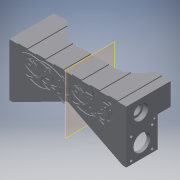
# Autodesk Inventor part: Crossmount
Saved by Autodesk Inventor 2016 (Build 200138000, 138)
## iProperties
Created: 2016-07-16
Part Number: Crossmount
Material: Generic
Document SubType Name: Modeling
Designer: Scott
Density: 1 g/cm^3
Appearance: Default
Author: Scott
Autodesk Inventor part; units mm, degrees
(part 1 of 2)
ref_plane "YZ Plane" through (0, 0, 0) normal (1, 0, 0) x (0, 1, 0)
ref_plane "XZ Plane" through (0, 0, 0) normal (0, 1, 0) x (-1, 0, 0)
ref_plane "XY Plane" through (0, 0, 0) normal (0, 0, 1) x (1, 0, 0)
sketch "Sketch1" plane through (0, 0, 0) normal (0, 0, 1) x (1, 0, 0)
  circle A0 centre (0, 0) radius 4 projected
  circle A1 centre (-152.4, 0) radius 4 projected
  circle A2 centre (0, 0) radius 10.16
  circle A3 centre (-152.4, 0) radius 10.16
  point P0 (0, 0)
  dimension "d0" = 20.32
  dimension "d1" = 20.32
  constraints: 2 centre point, 2 coincident
  measures "d0" diameter of A2
  measures "d1" diameter of A3
extrude "Extrusion1" add sketch "Sketch1" against normal blind 25.4
sketch "Sketch2" plane through (0, 0, 0) normal (0, 0, 1) x (1, 0, 0)
  circle A0 centre (-152.4, 0) radius 10.16 projected
  circle A1 centre (0, 0) radius 10.16 projected
  line L0 (10.16, -10.16) -> (-162.56, -10.16)
  line L1 (-162.56, -10.16) -> (-162.56, 10.16)
  line L2 (-162.56, 10.16) -> (10.16, 10.16)
  line L3 (10.16, 10.16) -> (10.16, -10.16)
  point P0 (0, 0)
  constraints: 8 end point, 2 parallel, 1 horizontal, 1 perpendicular
extrude "Extrusion2" add sketch "Sketch2" along normal blind 38.1
sketch "Sketch3" plane through (-162.56, -10.16, 0) normal (-1, 0, 0) x (0, 0, 1)
  circle A0 centre (18.605, 8.132) radius 4 projected
  line L0 (-0.445, -10.918) -> (37.655, -10.918)
  line L1 (37.655, -10.918) -> (37.655, 27.182)
  line L2 (37.655, 27.182) -> (-0.445, 27.182)
  line L3 (-0.445, 27.182) -> (-0.445, -10.918)
  line L4 (-0.445, -10.918) -> (37.655, 27.182) construction
  line L5 (37.655, -10.918) -> (-0.445, 27.182) construction
  point P0 (0, 10.16)
  dimension "d6" = 38.1
  dimension "d7" = 38.1
  constraints: 12 end point, 2 midpoint, 2 parallel, 1 horizontal, 1 perpendicular
  measures "d6" distance of L2.end L1.end
  measures "d7" distance of L1.end L0.end
extrude "Extrusion3" add sketch "Sketch3" against normal up to surface (172.72 mm away)
sketch "Sketch4" plane through (-162.56, -10.16, 38.1) normal (-1, 0, 0) x (0, 0, 1)
  circle A0 centre (-19.495, 8.132) radius 4 projected
  circle A1 centre (-19.495, 8.132) radius 11
  point P0 (-38.1, 10.16)
  dimension "d10" = 22
  constraints: 1 centre point, 1 coincident
  measures "d10" diameter of A1
extrude "Extrusion4" cut sketch "Sketch4" against normal blind 7 contours A0 | A1
sketch "Sketch5" plane through (-155.56, -2.028, 18.605) normal (-1, 0, 0) x (0, 0, 1)
  circle A0 centre (0, 0) radius 5 projected
  point P0 (-18.605, 2.028)
extrude "Extrusion5" cut sketch "Sketch5" against normal blind 214.9625
sketch "Sketch6" plane through (10.16, -10.16, 38.1) normal (1, 0, 0) x (0, 0, -1)
  circle A0 centre (19.495, 8.132) radius 5 projected
  line L0 (0.445, 20.32) -> (0, 20.32) projected
  line L1 (0, 0) -> (0, 20.32) projected
  line L2 (0.445, 0) -> (0, 0) projected
  line L3 (0.445, -10.918) -> (0.445, 0) projected
  line L4 (38.545, -10.918) -> (0.445, -10.918) projected
  line L5 (38.545, 10.16) -> (38.545, -10.918) projected
  line L6 (38.545, 27.182) -> (38.545, 10.16) projected
  line L7 (0.445, 27.182) -> (38.545, 27.182) projected
  line L8 (0.445, 20.32) -> (0.445, 27.182) projected
  circle A1 centre (19.495, 8.132) radius 11
  point P0 (38.1, 10.16)
  dimension "d15" = 22
  constraints: 1 centre point, 1 coincident
  measures "d15" diameter of A1
extrude "Extrusion6" cut sketch "Sketch6" against normal blind 7 contours A1
sketch "Sketch7" plane through (0, 0, -25.4) normal (0, 0, -1) x (-1, 0, 0)
  line L0 (-10.16, 17.022) -> (-10.16, 0) projected
  circle A0 centre (0, 0) radius 10.16 projected
  line L1 (-10.16, 0) -> (-10.16, -21.078) projected
  line L2 (162.56, -21.078) -> (-10.16, -21.078) projected
  line L3 (162.56, 0) -> (162.56, -21.078) projected
  circle A1 centre (152.4, 0) radius 10.16 projected
  line L4 (162.56, 17.022) -> (162.56, 0) projected
  line L5 (162.56, 17.022) -> (-10.16, 17.022) projected
  line L6 (162.56, 17.022) -> (-10.16, 17.022) projected
  line L7 (-10.16, -17.022) -> (10.16, -17.022)
  line L8 (10.16, -17.022) -> (10.16, 17.022)
  line L9 (10.16, 17.022) -> (-10.16, 17.022)
  line L10 (-10.16, 17.022) -> (-10.16, -17.022)
  line L11 (-10.16, -17.022) -> (10.16, 17.022) construction
  line L12 (10.16, -17.022) -> (-10.16, 17.022) construction
  point P0 (0, 0)
  constraints: 12 end point, 2 horizontal alignment, 2 midpoint, 2 parallel, 1 horizontal, 1 perpendicular, 1 point on line
extrude "Extrusion7" add sketch "Sketch7" against normal up to surface (24.955 mm away) contours L5 L8 A0 L0 | A0 L8 L7 L1
chamfer "Chamfer1" distance 24.892 angle 45 1 edges at (-10.16, 0, -0.445)
sketch "Sketch8" plane through (-152.4, 0, -25.4) normal (0, 0, -1) x (-1, 0, 0)
  circle A0 centre (0, 0) radius 4 projected
  circle A1 centre (0, 0) radius 10.16 projected
  line L0 (-117.348, -17.022) -> (-117.348, 17.022) projected
  line L1 (-117.348, -17.022) -> (-162.56, -17.022) projected
  line L2 (-162.56, -17.022) -> (-162.56, -21.078) projected
  line L3 (10.16, -21.078) -> (-162.56, -21.078) projected
  line L4 (10.16, 0) -> (10.16, -21.078) projected
  circle A2 centre (0, 0) radius 10.16 projected
  line L5 (10.16, 17.022) -> (10.16, 0) projected
  line L6 (10.16, 17.022) -> (-117.348, 17.022) projected
  line L7 (10.16, -17.022) -> (-10.16, -17.022)
  line L8 (-10.16, -17.022) -> (-10.16, 17.022)
  line L9 (-10.16, 17.022) -> (10.16, 17.022)
  line L10 (10.16, 17.022) -> (10.16, -17.022)
  line L11 (10.16, -17.022) -> (-10.16, 17.022) construction
  line L12 (-10.16, -17.022) -> (10.16, 17.022) construction
  point P0 (-152.4, 0)
  constraints: 12 end point, 2 midpoint, 2 parallel, 1 horizontal, 1 horizontal alignment, 1 perpendicular, 1 point on line
extrude "Extrusion8" add sketch "Sketch8" against normal up to surface (24.955 mm away) contours L4 L7 L8 A1 | A1 L8 L6 L5
chamfer "Chamfer2" distance 24.892 angle 45 1 edges at (-142.24, 0, -0.445)
sketch "Sketch9" plane through (-155.56, -2.028, 18.605) normal (-1, 0, 0) x (0, 0, 1)
  circle A0 centre (0, 0) radius 11 projected
  circle A1 centre (0, 0) radius 7.5
  point P0 (-18.605, 2.028)
  dimension "d28" = 15
  constraints: 1 centre point, 1 coincident
  measures "d28" diameter of A1
extrude "Extrusion9" cut sketch "Sketch9" against normal blind 219.725 contours A1
sketch "Sketch10" plane through (-162.56, -10.16, 38.1) normal (-1, 0, 0) x (0, 0, 1)
  circle A0 centre (-19.495, 8.132) radius 11 projected
  line L0 (-0.445, 0) -> (0, 0) projected
  line L1 (0, 20.32) -> (0, 0) projected
  line L2 (-0.445, 20.32) -> (0, 20.32) projected
  line L3 (-0.445, 20.32) -> (-0.445, 27.182) projected
  line L4 (-0.445, 27.182) -> (-63.5, 27.182) projected
  line L5 (-63.5, -6.862) -> (-63.5, 27.182) projected
  line L6 (-63.5, -6.862) -> (-38.545, -6.862) projected
  line L7 (-38.545, -6.862) -> (-38.545, -10.918) projected
  line L8 (-38.545, -10.918) -> (-0.445, -10.918) projected
  line L9 (-0.445, -10.918) -> (-0.445, 0) projected
  line L10 (-0.445, -10.918) -> (-41.445, -10.918)
  line L11 (-41.445, -10.918) -> (-41.445, -51.918)
  line L12 (-41.445, -51.918) -> (-0.445, -51.918)
  line L13 (-0.445, -51.918) -> (-0.445, -10.918)
  circle A1 centre (-20.945, -31.418) radius 12.5
  line L14 (-20.945, -31.418) -> (-20.945, -46.918)
  line L15 (-20.945, -46.918) -> (-5.445, -46.918)
  circle A2 centre (-5.445, -46.918) radius 2
  circle A3 centre (-36.445, -46.918) radius 2
  circle A4 centre (-5.445, -15.918) radius 2
  circle A5 centre (-36.445, -15.918) radius 2
  point P0 (-38.1, 10.16)
  dimension "d31" = 41
  dimension "d32" = 41
  dimension "d33" = 25
  dimension "d34" = 15.5
  dimension "d35" = 15.5
  dimension "d36" = 4
  dimension "d39" = 31
  dimension "d42" = 31
  constraints: 12 end point, 5 centre point, 3 parallel, 2 horizontal, 2 vertical, 1 coincident, 1 perpendicular, 6 other
  measures "d31" distance of L12.end L11.end
  measures "d32" distance of L11.end L10.end
  measures "d33" diameter of A1
  measures "d34" distance of L14.start L14.end
  measures "d35" distance of L14.end L15.end
  measures "d36" diameter of A2
  measures "d39" distance of A2.centre A3.centre
  measures "d42" distance of A2.centre A4.centre
extrude "Extrusion10" add sketch "Sketch10" against normal blind 5.08 contours L13 L12 L11 L10 L8
sketch "Sketch11" plane through (-162.56, -10.16, 37.655) normal (0, 0, 1) x (1, 0, 0)
  line L0 (0, 0) -> (172.72, 0) projected
  line L1 (0, -51.918) -> (0, 0) projected
  line L2 (0, -51.918) -> (5.08, -51.918) projected
  line L3 (5.08, -10.918) -> (5.08, -51.918) projected
  line L4 (5.08, -10.918) -> (172.72, -10.918) projected
  line L5 (172.72, -10.918) -> (172.72, 0) projected
  line L6 (0, -51.918) -> (5.08, -51.918) projected
  line L7 (5.08, -51.918) -> (86.36, -10.918)
  line L8 (5.08, -10.918) -> (172.72, -10.918) projected
  line L9 (86.36, -10.918) -> (172.72, -10.918)
  line L10 (172.72, 20.32) -> (172.72, 27.182) projected
  line L11 (172.72, -10.918) -> (172.72, 27.182)
  line L12 (172.72, 27.182) -> (0, 27.182)
  line L13 (0, -10.918) -> (0, -51.918) projected
  line L14 (0, 27.182) -> (0, -51.918)
  line L15 (5.08, -10.918) -> (5.08, -51.918) projected
  line L16 (0, -51.918) -> (5.08, -51.918)
  point P0 (162.56, 10.16)
  constraints: 12 end point, 4 perpendicular, 1 horizontal, 1 point on line
extrude "Extrusion11" add sketch "Sketch11" along normal blind 2.54
sketch "Sketch12" plane through (-157.48, -21.078, -0.445) normal (0, -1, 0) x (1, 0, 0)
  line L0 (0, 38.1) -> (0, 0) projected
  line L1 (0, 0) -> (167.64, 0) projected
  line L2 (167.64, 0) -> (167.64, 40.64) projected
  line L3 (81.28, 40.64) -> (167.64, 40.64) projected
  line L4 (81.28, 38.1) -> (81.28, 40.64) projected
  line L5 (0, 38.1) -> (81.28, 38.1) projected
  line L6 (167.64, 30.05) -> (167.64, 8.05) projected
  line L7 (167.64, 19.05) -> (-5.08, 18.87)
  line L8 (-5.08, -2.9) -> (-5.08, 40.64) projected
  line L9 (24.13, 31.66) -> (138.43, 31.66)
  line L10 (138.43, 31.66) -> (138.43, 6.26)
  line L11 (138.43, 6.26) -> (24.13, 6.26)
  line L12 (24.13, 6.26) -> (24.13, 31.66)
  line L13 (24.13, 31.66) -> (138.43, 6.26) construction
  line L14 (138.43, 31.66) -> (24.13, 6.26) construction
  point P0 (157.48, 0.445)
  point P1 (81.28, 18.96)
  dimension "d49" = 114.3
  dimension "d50" = 25.4
  constraints: 14 end point, 5 midpoint, 2 parallel, 1 horizontal, 1 perpendicular
  measures "d49" distance of L10.end L11.end
  measures "d50" distance of L9.end L10.end
extrude "Extrusion12" cut sketch "Sketch12" against normal blind 34.29 contours L12 L9 L10 L7 | L7 L10 L11 L12
sketch "Sketch13" plane through (-162.56, -62.078, -3.345) normal (0, 0, -1) x (-1, 0, 0)
  line L0 (0, 41) -> (0, 0) projected
  line L1 (0, 41) -> (-5.08, 41) projected
  line L2 (-5.08, 0) -> (-5.08, 41) projected
  line L3 (0, 0) -> (-5.08, 0) projected
  line L4 (-45.212, 79.1) -> (-45.212, 45.056) projected
  line L5 (-45.212, 79.1) -> (-127.508, 79.1) projected
  line L6 (-127.508, 45.056) -> (-127.508, 79.1) projected
  line L7 (-127.508, 45.056) -> (-172.72, 45.056) projected
  line L8 (-172.72, 45.056) -> (-172.72, 41) projected
  line L9 (-5.08, 41) -> (-172.72, 41) projected
  line L10 (0, 41) -> (-5.08, 41) projected
  line L11 (0, 45.056) -> (0, 41) projected
  line L12 (0, 45.056) -> (-45.212, 45.056) projected
  line L13 (-5.08, 0) -> (-5.08, 41) projected
  line L14 (-5.08, 0) -> (-38.8543, 45.056)
  point P0 (-162.56, 62.078)
  constraints: 2 end point, 1 point on line
extrude "Extrusion13" add sketch "Sketch13" along normal blind 2.54 contours L0 L3 L2 L1 | L1 L9 L14 L12 L11 | L2 L14 L9
ref_plane "Work Plane1" through (-76.2, -17.022, -25.4) normal (1, 0, 0) x (0, 0, -1)
mirror "Mirror1" about plane through (-76.2, -17.022, -25.4) normal (1, 0, 0) of "Extrusion10", "Extrusion11", "Extrusion12"
mirror "Mirror2" about plane through (-76.2, -17.022, -25.4) normal (1, 0, 0) of "Extrusion13"
sketch "Sketch14" plane through (-162.56, -10.16, 40.195) normal (0, 0, 1) x (1, 0, 0)
  line L0 (139.4566, -12.9778) -> (139.0497, -12.9778)
  spline S0 degree 2 poles (139.0497, -12.9778) (135.9425, -12.3859) (131.4297, -8.9458) knots 0 0 0 1 1 1
  spline S1 degree 2 poles (131.4297, -8.9458) (130.0611, -7.8361) (129.0993, -6.4305) knots 0 0 0 1 1 1
  spline S2 degree 2 poles (129.0993, -6.4305) (128.2115, -5.7647) (128.2115, -5.0619) knots 0 0 0 1 1 1
  line L1 (128.2115, -5.0619) -> (128.3225, -4.9509)
  line L2 (128.3225, -4.9509) -> (127.4347, -3.8782)
  line L3 (127.4347, -3.8782) -> (127.4347, -3.7672)
  spline S3 degree 2 poles (127.4347, -3.7672) (128.2485, -4.47) (128.6924, -4.47) knots 0 0 0 1 1 1
  line L4 (128.6924, -4.47) -> (128.9883, -4.47)
  spline S4 degree 2 poles (128.9883, -4.47) (130.283, -1.7697) (133.2792, 1.7074) knots 0 0 0 1 1 1
  spline S5 degree 2 poles (133.2792, 1.7074) (137.829, 5.7023) (139.8265, 5.7023) knots 0 0 0 1 1 1
  line L5 (139.8265, 5.7023) -> (139.8265, 12.4345)
  line L6 (139.8265, 12.4345) -> (140.0484, 12.4345)
  spline S6 degree 2 poles (140.0484, 12.4345) (140.7143, 9.8082) (141.4911, 9.8082) knots 0 0 0 1 1 1
  line L7 (141.4911, 9.8082) -> (142.8597, 9.6233)
  line L8 (142.8597, 9.6233) -> (143.3406, 9.6233)
  line L9 (143.3406, 9.6233) -> (143.3406, 13.3223)
  line L10 (143.3406, 13.3223) -> (139.5306, 15.1718)
  line L11 (139.5306, 15.1718) -> (139.5306, 15.3568)
  line L12 (139.5306, 15.3568) -> (142.1939, 15.3568)
  line L13 (142.1939, 15.3568) -> (142.5638, 15.4678)
  spline S7 degree 2 poles (142.5638, 15.4678) (143.7475, 15.3568) (143.7475, 15.1718) knots 0 0 0 1 1 1
  line L14 (143.7475, 15.1718) -> (143.9324, 14.9869)
  line L15 (143.9324, 14.9869) -> (144.5243, 14.9869)
  spline S8 degree 2 poles (144.5243, 14.9869) (148.1123, 14.9869) (148.8151, 16.1336) knots 0 0 0 1 1 1
  spline S9 degree 2 poles (148.8151, 16.1336) (149.333, 16.7254) (149.333, 17.6872) knots 0 0 0 1 1 1
  spline S10 degree 2 poles (149.333, 17.6872) (149.333, 18.6859) (148.0383, 18.6859) knots 0 0 0 1 1 1
  line L16 (148.0383, 18.6859) -> (147.3725, 18.7599)
  line L17 (147.3725, 18.7599) -> (147.3725, 18.9818)
  spline S11 degree 2 poles (147.3725, 18.9818) (149.148, 18.9818) (151.7374, 17.5022) knots 0 0 0 1 1 1
  spline S12 degree 2 poles (151.7374, 17.5022) (153.032, 23.3837) (153.6239, 25.3072) knots 0 0 0 1 1 1
  line L18 (153.6239, 25.3072) -> (153.8088, 25.3072)
  spline S13 degree 2 poles (153.8088, 25.3072) (153.143, 19.1298) (152.5142, 16.4295) knots 0 0 0 1 1 1
  spline S14 degree 2 poles (152.5142, 16.4295) (151.5154, 13.4703) (148.9261, 9.6233) knots 0 0 0 1 1 1
  line L19 (148.9261, 9.6233) -> (149.333, 9.6233)
  spline S15 degree 2 poles (149.333, 9.6233) (150.8866, 9.6233) (150.8866, 9.9932) knots 0 0 0 1 1 1
  line L20 (150.8866, 9.9932) -> (151.3675, 12.0646)
  line L21 (151.3675, 12.0646) -> (151.5524, 12.0646)
  line L22 (151.5524, 12.0646) -> (151.5524, 4.4446)
  line L23 (151.5524, 4.4446) -> (151.3675, 4.4446)
  line L24 (151.3675, 4.4446) -> (151.3675, 4.8146)
  spline S16 degree 2 poles (151.3675, 4.8146) (151.3675, 5.7763) (150.1838, 6.4791) knots 0 0 0 1 1 1
  line L25 (150.1838, 6.4791) -> (147.5575, 6.4791)
  line L26 (147.5575, 6.4791) -> (147.5575, 5.7763)
  line L27 (147.5575, 5.7763) -> (147.6684, 2.8541)
  spline S17 degree 2 poles (147.6684, 2.8541) (147.5945, 2.2622) (147.4465, 2.2622) knots 0 0 0 1 1 1
  line L28 (147.4465, 2.2622) -> (147.5575, 0.8196)
  line L29 (147.5575, 0.8196) -> (147.5575, -2.1026)
  spline S18 degree 2 poles (147.5575, -2.1026) (147.5575, -2.2506) (146.1888, -2.6945) knots 0 0 0 1 1 1
  line L30 (146.1888, -2.6945) -> (145.8189, -3.5822)
  spline S19 degree 2 poles (145.8189, -3.5822) (145.8189, -4.655) (147.1506, -4.8399) knots 0 0 0 1 1 1
  spline S20 degree 2 poles (147.1506, -4.8399) (148.4082, -4.8399) (150.1098, -3.2863) knots 0 0 0 1 1 1
  spline S21 degree 2 poles (150.1098, -3.2863) (151.7374, -2.3246) (154.4746, 1.1895) knots 0 0 0 1 1 1
  spline S22 degree 2 poles (154.4746, 1.1895) (155.0665, 2.6321) (155.9543, 6.2942) knots 0 0 0 1 1 1
  line L31 (155.9543, 6.2942) -> (156.1392, 6.2942)
  spline S23 degree 2 poles (156.1392, 6.2942) (155.6213, 1.7074) (154.4007, 0.2278) knots 0 0 0 1 1 1
  spline S24 degree 2 poles (154.4007, 0.2278) (153.032, -1.6588) (151.3675, -3.3973) knots 0 0 0 1 1 1
  spline S25 degree 2 poles (151.3675, -3.3973) (149.296, -5.8756) (147.4465, -6.6154) knots 0 0 0 1 1 1
  spline S26 degree 2 poles (147.4465, -6.6154) (142.2309, -8.7609) (136.4234, -8.7609) knots 0 0 0 1 1 1
  spline S27 degree 2 poles (136.4234, -8.7609) (134.2779, -8.6499) (132.9093, -8.391) knots 0 0 0 1 1 1
  line L32 (132.9093, -8.391) -> (132.7983, -8.391)
  line L33 (132.7983, -8.391) -> (132.7983, -8.465)
  spline S28 degree 2 poles (132.7983, -8.465) (132.9833, -8.465) (134.2779, -9.7226) knots 0 0 0 1 1 1
  line L34 (134.2779, -9.7226) -> (136.9043, -11.3872)
  spline S29 degree 2 poles (136.9043, -11.3872) (138.051, -12.09) (140.2334, -12.5709) knots 0 0 0 1 1 1
  line L35 (140.2334, -12.5709) -> (140.2334, -12.6819)
  line L36 (140.2334, -12.6819) -> (139.4566, -12.9778)
  line L37 (143.2666, -2.6205) -> (143.2666, 2.4842)
  spline S30 degree 2 poles (143.2666, 2.4842) (142.9337, 2.3732) (141.713, 1.0046) knots 0 0 0 1 1 1
  line L38 (141.713, 1.0046) -> (141.8979, 1.0046)
  line L39 (141.8979, 1.0046) -> (141.8979, 0.9306)
  spline S31 degree 2 poles (141.8979, 0.9306) (134.8328, -3.9891) (134.4629, -4.47) knots 0 0 0 1 1 1
  line L40 (134.4629, -4.47) -> (133.7971, -5.3578)
  spline S32 degree 2 poles (133.7971, -5.3578) (135.3507, -7.2813) (136.7193, -7.2813) knots 0 0 0 1 1 1
  line L41 (136.7193, -7.2813) -> (137.977, -7.3922)
  spline S33 degree 2 poles (137.977, -7.3922) (141.676, -7.3922) (142.8597, -4.7659) knots 0 0 0 1 1 1
  spline S34 degree 2 poles (142.8597, -4.7659) (143.2666, -4.0261) (143.2666, -2.6205) knots 0 0 0 1 1 1
  line L42 (143.3406, 4.9255) -> (143.3406, 6.4791)
  line L43 (143.3406, 6.4791) -> (143.2666, 6.4791)
  spline S35 degree 2 poles (143.2666, 6.4791) (141.0472, 6.3681) (140.8992, 5.8873) knots 0 0 0 1 1 1
  line L44 (140.8992, 5.8873) -> (140.8992, 5.7763)
  line L45 (140.8992, 5.7763) -> (142.5638, 6.0722)
  line L46 (142.5638, 6.0722) -> (142.5638, 5.8873)
  spline S36 degree 2 poles (142.5638, 5.8873) (140.4183, 5.4804) (140.4183, 4.9995) knots 0 0 0 1 1 1
  line L47 (140.4183, 4.9995) -> (140.0484, 3.6309)
  line L48 (140.0484, 3.6309) -> (139.8265, 3.6309)
  line L49 (139.8265, 3.6309) -> (139.8265, 5.1105)
  spline S37 degree 2 poles (139.8265, 5.1105) (137.1632, 5.1105) (132.9833, 0.1168) knots 0 0 0 1 1 1
  line L50 (132.9833, 0.1168) -> (131.5407, -2.0287)
  line L51 (131.5407, -2.0287) -> (130.6529, -3.4713)
  line L52 (130.6529, -3.4713) -> (130.7639, -3.4713)
  spline S38 degree 2 poles (130.7639, -3.4713) (134.2779, -1.2519) (135.9425, -0.771) knots 0 0 0 1 1 1
  spline S39 degree 2 poles (135.9425, -0.771) (138.9387, 0.9676) (141.3061, 3.261) knots 0 0 0 1 1 1
  spline S40 degree 2 poles (141.3061, 3.261) (142.8967, 4.8515) (143.3406, 4.9255) knots 0 0 0 1 1 1
  spline S41 degree 2 poles (147.7424, 9.9932) (149.9618, 12.6195) (150.7756, 14.469) knots 0 0 0 1 1 1
  line L53 (150.7756, 14.469) -> (150.6646, 14.469)
  spline S42 degree 2 poles (150.6646, 14.469) (150.1098, 14.0991) (148.3343, 13.5073) knots 0 0 0 1 1 1
  spline S43 degree 2 poles (148.3343, 13.5073) (147.6684, 12.9524) (147.6684, 11.8427) knots 0 0 0 1 1 1
  line L54 (147.6684, 11.8427) -> (147.6684, 9.9932)
  line L55 (147.6684, 9.9932) -> (147.7424, 9.9932)
  line L56 (147.0766, 18.8709) -> (146.7807, 18.8709)
  line L57 (146.7807, 18.8709) -> (146.7807, 19.0928)
  line L58 (146.7807, 19.0928) -> (147.0766, 19.0928)
  line L59 (147.0766, 19.0928) -> (147.0766, 18.8709)
  line L60 (124.8824, -8.8719) -> (112.7496, -8.8719)
  line L61 (112.7496, -8.8719) -> (112.7496, -8.7609)
  spline S44 degree 2 poles (112.7496, -8.7609) (113.8593, -7.9471) (116.0787, -6.9114) knots 0 0 0 1 1 1
  spline S45 degree 2 poles (116.0787, -6.9114) (116.6706, -5.2468) (116.6706, -4.1741) knots 0 0 0 1 1 1
  line L62 (116.6706, -4.1741) -> (116.6706, 7.5518)
  spline S46 degree 2 poles (116.6706, 7.5518) (115.2649, 7.5518) (114.895, 6.3681) knots 0 0 0 1 1 1
  line L63 (114.895, 6.3681) -> (114.7101, 6.5901)
  line L64 (114.7101, 6.5901) -> (114.5251, 6.5901)
  line L65 (114.5251, 6.5901) -> (114.5251, 12.1386)
  line L66 (114.5251, 12.1386) -> (114.7101, 12.1386)
  spline S47 degree 2 poles (114.7101, 12.1386) (115.117, 10.2891) (115.9678, 10.2891) knots 0 0 0 1 1 1
  line L67 (115.9678, 10.2891) -> (116.6706, 10.2891)
  line L68 (116.6706, 10.2891) -> (116.6706, 13.2113)
  spline S48 degree 2 poles (116.6706, 13.2113) (116.6706, 13.9881) (113.9333, 14.7649) knots 0 0 0 1 1 1
  spline S49 degree 2 poles (113.9333, 14.7649) (113.9333, 14.9869) (113.3414, 14.9869) knots 0 0 0 1 1 1
  line L69 (113.3414, 14.9869) -> (113.3414, 15.1718)
  line L70 (113.3414, 15.1718) -> (124.1796, 15.1718)
  spline S50 degree 2 poles (124.1796, 15.1718) (123.6987, 18.8709) (122.626, 21.1273) knots 0 0 0 1 1 1
  spline S51 degree 2 poles (122.626, 21.1273) (122.1451, 23.2357) (121.1464, 25.825) knots 0 0 0 1 1 1
  line L71 (121.1464, 25.825) -> (121.0724, 26.3799)
  line L72 (121.0724, 26.3799) -> (121.1464, 26.4909)
  line L73 (121.1464, 26.4909) -> (121.2574, 26.4909)
  spline S52 degree 2 poles (121.2574, 26.4909) (124.8824, 18.8709) (124.8824, 16.2445) knots 0 0 0 1 1 1
  line L74 (124.8824, 16.2445) -> (124.9564, 15.5417)
  line L75 (124.9564, 15.5417) -> (124.9564, 13.5073)
  spline S53 degree 2 poles (124.9564, 13.5073) (124.9564, 2.8911) (121.1464, -5.0619) knots 0 0 0 1 1 1
  spline S54 degree 2 poles (121.1464, -5.0619) (121.4793, -7.0223) (122.1451, -7.0223) knots 0 0 0 1 1 1
  spline S55 degree 2 poles (122.1451, -7.0223) (122.737, -7.5032) (124.8824, -8.6499) knots 0 0 0 1 1 1
  line L76 (124.8824, -8.6499) -> (124.8824, -8.8719)
  line L77 (124.1796, 13.6182) -> (124.1796, 15.0979)
  spline S56 degree 2 poles (124.1796, 15.0979) (122.0342, 15.0979) (121.2574, 13.0264) knots 0 0 0 1 1 1
  line L78 (121.2574, 13.0264) -> (120.8505, 11.0659)
  line L79 (120.8505, 11.0659) -> (120.8505, 10.2891)
  line L80 (120.8505, 10.2891) -> (122.4411, 10.2891)
  spline S57 degree 2 poles (122.4411, 10.2891) (122.7, 10.2891) (122.9219, 11.8427) knots 0 0 0 1 1 1
  line L81 (122.9219, 11.8427) -> (123.1069, 11.8427)
  line L82 (123.1069, 11.8427) -> (123.1069, 6.3681)
  line L83 (123.1069, 6.3681) -> (122.9219, 6.3681)
  spline S58 degree 2 poles (122.9219, 6.3681) (122.9219, 7.2929) (121.8492, 7.5518) knots 0 0 0 1 1 1
  line L84 (121.8492, 7.5518) -> (120.9614, 7.5518)
  line L85 (120.9614, 7.5518) -> (120.9614, 1.0046)
  line L86 (120.9614, 1.0046) -> (120.7765, 0.8196)
  spline S59 degree 2 poles (120.7765, 0.8196) (120.7025, 1.1155) (119.9627, 1.1155) knots 0 0 0 1 1 1
  spline S60 degree 2 poles (119.9627, 1.1155) (119.0749, 1.1155) (118.89, -0.1421) knots 0 0 0 1 1 1
  spline S61 degree 2 poles (118.89, -0.1421) (118.89, -1.0669) (120.1846, -1.2519) knots 0 0 0 1 1 1
  spline S62 degree 2 poles (120.1846, -1.2519) (121.2944, -1.2519) (121.5533, 1.4854) knots 0 0 0 1 1 1
  spline S63 degree 2 poles (121.5533, 1.4854) (123.5138, 6.1462) (123.5138, 8.4396) knots 0 0 0 1 1 1
  line L87 (123.5138, 8.4396) -> (124.1796, 13.6182)
  line L88 (116.4116, -12.6819) -> (114.3402, -12.6819)
  spline S64 degree 2 poles (114.3402, -12.6819) (103.0212, -12.6819) (94.3284, -8.206) knots 0 0 0 1 1 1
  line L89 (94.3284, -8.206) -> (92.8488, -8.0951)
  spline S65 degree 2 poles (92.8488, -8.0951) (91.6281, -8.0951) (88.484, -8.6869) knots 0 0 0 1 1 1
  spline S66 degree 2 poles (88.484, -8.6869) (91.1103, -5.9496) (93.6256, -2.7315) knots 0 0 0 1 1 1
  line L90 (93.6256, -2.7315) -> (93.6256, -3.9891)
  spline S67 degree 2 poles (93.6256, -3.9891) (93.6256, -6.2455) (97.4726, -6.8374) knots 0 0 0 1 1 1
  spline S68 degree 2 poles (97.4726, -6.8374) (104.0569, -5.0619) (104.2788, -4.692) knots 0 0 0 1 1 1
  spline S69 degree 2 poles (104.2788, -4.692) (105.5735, -4.1741) (105.5735, -3.3973) knots 0 0 0 1 1 1
  spline S70 degree 2 poles (105.5735, -3.3973) (105.5735, -2.4725) (104.3898, -2.1396) knots 0 0 0 1 1 1
  line L91 (104.3898, -2.1396) -> (101.0607, -3.3973)
  spline S71 degree 2 poles (101.0607, -3.3973) (98.0645, -2.5465) (94.0325, 0.1168) knots 0 0 0 1 1 1
  spline S72 degree 2 poles (94.0325, 0.1168) (90.4075, 2.928) (90.4075, 4.9995) knots 0 0 0 1 1 1
  line L92 (90.4075, 4.9995) -> (89.8526, 6.738)
  spline S73 degree 2 poles (89.8526, 6.738) (89.8526, 12.2866) (103.9089, 18.8339) knots 0 0 0 1 1 1
  line L93 (103.9089, 18.8339) -> (104.0199, 18.8339)
  line L94 (104.0199, 18.8339) -> (98.6193, 15.2458)
  line L95 (98.6193, 15.2458) -> (98.6193, 15.1348)
  line L96 (98.6193, 15.1348) -> (99.0262, 15.2458)
  spline S74 degree 2 poles (99.0262, 15.2458) (101.2826, 15.2458) (104.3898, 12.6195) knots 0 0 0 1 1 1
  spline S75 degree 2 poles (104.3898, 12.6195) (106.0544, 14.2471) (106.0544, 14.7649) knots 0 0 0 1 1 1
  line L97 (106.0544, 14.7649) -> (104.4638, 16.6884)
  line L98 (104.4638, 16.6884) -> (104.4638, 16.7994)
  line L99 (104.4638, 16.7994) -> (110.3822, 12.2496)
  line L100 (110.3822, 12.2496) -> (110.3082, 12.2496)
  spline S76 degree 2 poles (110.3082, 12.2496) (109.6424, 12.6565) (109.1246, 12.6565) knots 0 0 0 1 1 1
  line L101 (109.1246, 12.6565) -> (108.2368, 12.6565)
  line L102 (108.2368, 12.6565) -> (106.6092, 10.696)
  line L103 (106.6092, 10.696) -> (106.6092, 10.622)
  spline S77 degree 2 poles (106.6092, 10.622) (110.1233, 5.4434) (111.122, 2.928) knots 0 0 0 1 1 1
  spline S78 degree 2 poles (111.122, 2.928) (108.5327, 6.3681) (105.7214, 9.7343) knots 0 0 0 1 1 1
  spline S79 degree 2 poles (105.7214, 9.7343) (103.465, 7.1079) (103.465, 6.2942) knots 0 0 0 1 1 1
  line L104 (103.465, 6.2942) -> (104.9077, 3.8528)
  line L105 (104.9077, 3.8528) -> (104.8337, 3.8528)
  line L106 (104.8337, 3.8528) -> (97.6576, 9.4753)
  line L107 (97.6576, 9.4753) -> (97.7315, 9.4753)
  line L108 (97.7315, 9.4753) -> (100.2839, 8.4026)
  line L109 (100.2839, 8.4026) -> (100.3948, 8.4026)
  spline S80 degree 2 poles (100.3948, 8.4026) (101.0977, 8.4026) (103.3911, 11.4358) knots 0 0 0 1 1 1
  spline S81 degree 2 poles (103.3911, 11.4358) (101.6525, 12.5085) (100.9867, 12.5085) knots 0 0 0 1 1 1
  line L110 (100.9867, 12.5085) -> (100.7647, 12.5085)
  spline S82 degree 2 poles (100.7647, 12.5085) (97.2507, 12.5085) (93.1447, 6.3681) knots 0 0 0 1 1 1
  line L111 (93.1447, 6.3681) -> (93.1447, 6.2572)
  spline S83 degree 2 poles (93.1447, 6.2572) (95.1792, 3.7048) (97.3616, 2.6321) knots 0 0 0 1 1 1
  spline S84 degree 2 poles (97.3616, 2.6321) (99.692, 1.2635) (103.613, 0.1908) knots 0 0 0 1 1 1
  spline S85 degree 2 poles (103.613, 0.1908) (106.0174, -0.9559) (106.9421, -0.9559) knots 0 0 0 1 1 1
  line L112 (106.9421, -0.9559) -> (107.9039, -0.9559)
  spline S86 degree 2 poles (107.9039, -0.9559) (109.4575, -0.9559) (112.0838, 0.4127) knots 0 0 0 1 1 1
  spline S87 degree 2 poles (112.0838, 0.4127) (109.3835, -2.1026) (109.3835, -2.3246) knots 0 0 0 1 1 1
  line L113 (109.3835, -2.3246) -> (109.3835, -2.4355)
  line L114 (109.3835, -2.4355) -> (109.4575, -2.4355)
  spline S88 degree 2 poles (109.4575, -2.4355) (111.307, -1.8437) (114.932, 1.0785) knots 0 0 0 1 1 1
  spline S89 degree 2 poles (114.932, 1.0785) (116.1157, 1.4854) (118.853, 4.1117) knots 0 0 0 1 1 1
  spline S90 degree 2 poles (118.853, 4.1117) (119.5928, 5.3324) (120.4066, 6.1462) knots 0 0 0 1 1 1
  line L115 (120.4066, 6.1462) -> (123.5138, 11.7317)
  spline S91 degree 2 poles (123.5138, 11.7317) (123.5138, 12.2126) (124.8824, 13.7662) knots 0 0 0 1 1 1
  line L116 (124.8824, 13.7662) -> (124.9934, 13.7662)
  line L117 (124.9934, 13.7662) -> (124.9934, 13.6922)
  spline S92 degree 2 poles (124.9934, 13.6922) (121.1464, 4.7036) (119.3339, 3.4459) knots 0 0 0 1 1 1
  spline S93 degree 2 poles (119.3339, 3.4459) (113.2305, -2.3986) (110.2713, -3.8042) knots 0 0 0 1 1 1
  spline S94 degree 2 poles (110.2713, -3.8042) (106.7202, -5.9496) (100.9867, -8.391) knots 0 0 0 1 1 1
  line L118 (100.9867, -8.391) -> (100.1729, -8.5759)
  spline S95 degree 2 poles (100.1729, -8.5759) (100.2469, -8.7979) (103.3911, -9.6487) knots 0 0 0 1 1 1
  spline S96 degree 2 poles (103.3911, -9.6487) (107.312, -11.4242) (111.6399, -11.4242) knots 0 0 0 1 1 1
  spline S97 degree 2 poles (111.6399, -11.4242) (111.9728, -11.6831) (114.4512, -11.9051) knots 0 0 0 1 1 1
  line L119 (114.4512, -11.9051) -> (116.0047, -11.9051)
  spline S98 degree 2 poles (116.0047, -11.9051) (119.7038, -11.4242) (121.6643, -10.4624) knots 0 0 0 1 1 1
  spline S99 degree 2 poles (121.6643, -10.4624) (124.1056, -9.8706) (126.362, -8.9828) knots 0 0 0 1 1 1
  line L120 (126.362, -8.9828) -> (127.5457, -8.6869)
  line L121 (127.5457, -8.6869) -> (127.6567, -8.7979)
  line L122 (127.6567, -8.7979) -> (127.6567, -8.8719)
  spline S100 degree 2 poles (127.6567, -8.8719) (119.6298, -12.6079) (117.1884, -12.6079) knots 0 0 0 1 1 1
  line L123 (117.1884, -12.6079) -> (116.4116, -12.6819)
  spline S101 degree 2 poles (82.2696, -15.0492) (78.9035, -14.6793) (72.8741, -9.9076) knots 0 0 0 1 1 1
  spline S102 degree 2 poles (72.8741, -9.9076) (72.6891, -9.2048) (71.2095, -7.8361) knots 0 0 0 1 1 1
  spline S103 degree 2 poles (71.2095, -7.8361) (70.0258, -5.8387) (70.0258, -5.5057) knots 0 0 0 1 1 1
  line L124 (70.0258, -5.5057) -> (69.9518, -4.1001)
  spline S104 degree 2 poles (69.9518, -4.1001) (70.3217, -3.9521) (71.0246, -1.7697) knots 0 0 0 1 1 1
  spline S105 degree 2 poles (71.0246, -1.7697) (71.8383, -0.9559) (73.281, 1.1525) knots 0 0 0 1 1 1
  spline S106 degree 2 poles (73.281, 1.1525) (74.4646, 2.6321) (75.3154, 2.6321) knots 0 0 0 1 1 1
  line L125 (75.3154, 2.6321) -> (75.4264, 2.3362)
  spline S107 degree 2 poles (75.4264, 2.3362) (75.3524, 1.4484) (75.2045, 1.4484) knots 0 0 0 1 1 1
  line L126 (75.2045, 1.4484) -> (75.2045, 1.2635)
  line L127 (75.2045, 1.2635) -> (75.3154, 1.2635)
  line L128 (75.3154, 1.2635) -> (75.2045, -0.697)
  line L129 (75.2045, -0.697) -> (75.2045, -1.1779)
  line L130 (75.2045, -1.1779) -> (75.7223, -3.5453)
  line L131 (75.7223, -3.5453) -> (75.4264, -3.8412)
  line L132 (75.4264, -3.8412) -> (75.2045, -3.8412)
  line L133 (75.2045, -3.8412) -> (75.1305, -3.7302)
  line L134 (75.1305, -3.7302) -> (75.0195, -3.7302)
  line L135 (75.0195, -3.7302) -> (75.1305, -3.6192)
  line L136 (75.1305, -3.6192) -> (75.1305, -3.5453)
  spline S108 degree 2 poles (75.1305, -3.5453) (75.1305, -2.6575) (74.0578, -2.1766) knots 0 0 0 1 1 1
  line L137 (74.0578, -2.1766) -> (73.6509, -2.1766)
  line L138 (73.6509, -2.1766) -> (73.281, -2.2876)
  line L139 (73.281, -2.2876) -> (73.17, -2.1766)
  line L140 (73.17, -2.1766) -> (73.059, -2.1766)
  spline S109 degree 2 poles (73.059, -2.1766) (72.2082, -2.1766) (71.4314, -4.2111) knots 0 0 0 1 1 1
  line L141 (71.4314, -4.2111) -> (71.4314, -4.9139)
  spline S110 degree 2 poles (71.4314, -4.9139) (71.4314, -6.0976) (73.7618, -6.7634) knots 0 0 0 1 1 1
  spline S111 degree 2 poles (73.7618, -6.7634) (74.9455, -6.4305) (76.5731, -5.2838) knots 0 0 0 1 1 1
  spline S112 degree 2 poles (76.5731, -5.2838) (78.3116, -3.9152) (79.6063, -1.1779) knots 0 0 0 1 1 1
  spline S113 degree 2 poles (79.6063, -1.1779) (80.901, 1.4484) (80.901, 4.1857) knots 0 0 0 1 1 1
  spline S114 degree 2 poles (80.901, 4.1857) (80.901, 8.2916) (78.4596, 11.6947) knots 0 0 0 1 1 1
  spline S115 degree 2 poles (78.4596, 11.6947) (77.6458, 10.3261) (77.6458, 9.6603) knots 0 0 0 1 1 1
  spline S116 degree 2 poles (77.6458, 9.6603) (78.4596, 8.3656) (78.4596, 8.1067) knots 0 0 0 1 1 1
  line L142 (78.4596, 8.1067) -> (78.3486, 8.1067)
  spline S117 degree 2 poles (78.3486, 8.1067) (74.7236, 9.8822) (73.6509, 10.622) knots 0 0 0 1 1 1
  line L143 (73.6509, 10.622) -> (73.6509, 10.733)
  line L144 (73.6509, 10.733) -> (75.4264, 10.733)
  spline S118 degree 2 poles (75.4264, 10.733) (76.2402, 11.4728) (76.98, 13.3593) knots 0 0 0 1 1 1
  spline S119 degree 2 poles (76.98, 13.3593) (75.0565, 15.5047) (66.8077, 18.9448) knots 0 0 0 1 1 1
  spline S120 degree 2 poles (66.8077, 18.9448) (66.1418, 18.9448) (61.0742, 20.7944) knots 0 0 0 1 1 1
  line L145 (61.0742, 20.7944) -> (59.5946, 21.0903)
  line L146 (59.5946, 21.0903) -> (59.1877, 20.9793)
  line L147 (59.1877, 20.9793) -> (58.1149, 21.2752)
  line L148 (58.1149, 21.2752) -> (57.819, 21.1643)
  line L149 (57.819, 21.1643) -> (57.2642, 21.2752)
  line L150 (57.2642, 21.2752) -> (57.1532, 21.1643)
  line L151 (57.1532, 21.1643) -> (57.0422, 21.1643)
  spline S121 degree 2 poles (57.0422, 21.1643) (55.5256, 21.5712) (52.9733, 21.8671) knots 0 0 0 1 1 1
  line L152 (52.9733, 21.8671) -> (52.5664, 21.7561)
  line L153 (52.5664, 21.7561) -> (52.2705, 21.8671)
  spline S122 degree 2 poles (52.2705, 21.8671) (51.0128, 21.7561) (49.5332, 21.3492) knots 0 0 0 1 1 1
  line L154 (49.5332, 21.3492) -> (49.4222, 21.4602)
  line L155 (49.4222, 21.4602) -> (49.3482, 21.4602)
  line L156 (49.3482, 21.4602) -> (43.6517, 19.7216)
  spline S123 degree 2 poles (43.6517, 19.7216) (42.1351, 19.0188) (40.0637, 18.6489) knots 0 0 0 1 1 1
  line L157 (40.0637, 18.6489) -> (40.0637, 18.8339)
  spline S124 degree 2 poles (40.0637, 18.8339) (48.1646, 22.4589) (49.9401, 22.4589) knots 0 0 0 1 1 1
  line L158 (49.9401, 22.4589) -> (51.3827, 22.6439)
  line L159 (51.3827, 22.6439) -> (53.4542, 22.6439)
  spline S125 degree 2 poles (53.4542, 22.6439) (64.8842, 22.6439) (73.6509, 18.0571) knots 0 0 0 1 1 1
  spline S126 degree 2 poles (73.6509, 18.0571) (75.1305, 17.4652) (78.2377, 15.8007) knots 0 0 0 1 1 1
  line L160 (78.2377, 15.8007) -> (78.3486, 15.8007)
  spline S127 degree 2 poles (78.3486, 15.8007) (78.3486, 16.0596) (79.0514, 17.1693) knots 0 0 0 1 1 1
  line L161 (79.0514, 17.1693) -> (77.7568, 18.7229)
  line L162 (77.7568, 18.7229) -> (77.9787, 18.7229)
  spline S128 degree 2 poles (77.9787, 18.7229) (82.2326, 16.5405) (82.3436, 16.2815) knots 0 0 0 1 1 1
  line L163 (82.3436, 16.2815) -> (82.2696, 16.2076)
  line L164 (82.2696, 16.2076) -> (82.1586, 16.2076)
  line L165 (82.1586, 16.2076) -> (81.3818, 16.3925)
  line L166 (81.3818, 16.3925) -> (81.2709, 16.3925)
  spline S129 degree 2 poles (81.2709, 16.3925) (80.4941, 16.0966) (80.0132, 14.8389) knots 0 0 0 1 1 1
  line L167 (80.0132, 14.8389) -> (79.9022, 14.432)
  spline S130 degree 2 poles (79.9022, 14.432) (81.7517, 13.2113) (82.7505, 11.3988) knots 0 0 0 1 1 1
  spline S131 degree 2 poles (82.7505, 11.3988) (85.4878, 7.2929) (85.4878, 2.0403) knots 0 0 0 1 1 1
  line L168 (85.4878, 2.0403) -> (85.4878, 1.7444)
  line L169 (85.4878, 1.7444) -> (85.2658, 0.0798)
  line L170 (85.2658, 0.0798) -> (84.711, 0.0798)
  line L171 (84.711, 0.0798) -> (84.6, 0.1908)
  spline S132 degree 2 poles (84.6, 0.1908) (83.0464, -0.1421) (83.0464, -1.2888) knots 0 0 0 1 1 1
  spline S133 degree 2 poles (83.0464, -1.2888) (83.0464, -2.3986) (84.3041, -2.8424) knots 0 0 0 1 1 1
  spline S134 degree 2 poles (84.3041, -2.8424) (89.2608, -1.3628) (91.4432, 2.0403) knots 0 0 0 1 1 1
  line L172 (91.4432, 2.0403) -> (92.109, 3.2979)
  line L173 (92.109, 3.2979) -> (92.331, 2.7061)
  line L174 (92.331, 2.7061) -> (92.331, 2.6321)
  spline S135 degree 2 poles (92.331, 2.6321) (91.8131, 0.0798) (86.1536, -4.2111) knots 0 0 0 1 1 1
  spline S136 degree 2 poles (86.1536, -4.2111) (82.3436, -6.7634) (80.3091, -7.5402) knots 0 0 0 1 1 1
  line L175 (80.3091, -7.5402) -> (79.4213, -8.0211)
  line L176 (79.4213, -8.0211) -> (79.3104, -8.1321)
  line L177 (79.3104, -8.1321) -> (78.9405, -8.0211)
  spline S137 degree 2 poles (78.9405, -8.0211) (77.9787, -8.317) (75.7223, -8.502) knots 0 0 0 1 1 1
  line L178 (75.7223, -8.502) -> (75.4264, -8.428)
  line L179 (75.4264, -8.428) -> (74.9455, -8.502)
  line L180 (74.9455, -8.502) -> (74.3537, -8.502)
  line L181 (74.3537, -8.502) -> (73.8728, -8.428)
  spline S138 degree 2 poles (73.8728, -8.428) (75.9443, -11.1653) (78.5336, -12.6079) knots 0 0 0 1 1 1
  spline S139 degree 2 poles (78.5336, -12.6079) (79.9762, -13.9025) (83.0464, -14.5684) knots 0 0 0 1 1 1
  line L182 (83.0464, -14.5684) -> (83.0464, -14.6793)
  line L183 (83.0464, -14.6793) -> (82.2696, -15.0492)
  spline S140 degree 2 poles (59.5206, -9.3897) (54.4529, -9.0198) (47.6837, -4.0261) knots 0 0 0 1 1 1
  spline S141 degree 2 poles (47.6837, -4.0261) (46.648, -4.2851) (44.5765, -5.2838) knots 0 0 0 1 1 1
  line L184 (44.5765, -5.2838) -> (44.5765, -5.0988)
  spline S142 degree 2 poles (44.5765, -5.0988) (46.7219, -3.6932) (47.9796, 0.5607) knots 0 0 0 1 1 1
  line L185 (47.9796, 0.5607) -> (48.3865, 2.7061)
  line L186 (48.3865, 2.7061) -> (48.5714, 2.7061)
  spline S143 degree 2 poles (48.5714, 2.7061) (49.1263, -1.7697) (50.0511, -1.7697) knots 0 0 0 1 1 1
  spline S144 degree 2 poles (50.0511, -1.7697) (51.2717, -2.9534) (53.5651, -2.9534) knots 0 0 0 1 1 1
  spline S145 degree 2 poles (53.5651, -2.9534) (57.0422, -2.9534) (59.4096, 1.8553) knots 0 0 0 1 1 1
  line L187 (59.4096, 1.8553) -> (59.3356, 1.9293)
  line L188 (59.3356, 1.9293) -> (51.1238, 1.9293)
  line L189 (51.1238, 1.9293) -> (53.1582, 5.7393)
  line L190 (53.1582, 5.7393) -> (53.8611, 7.1079)
  line L191 (53.8611, 7.1079) -> (54.046, 7.1079)
  line L192 (54.046, 7.1079) -> (53.972, 5.9612)
  line L193 (53.972, 5.9612) -> (53.972, 5.3324)
  spline S146 degree 2 poles (53.972, 5.3324) (54.157, 3.4089) (55.2297, 3.4089) knots 0 0 0 1 1 1
  line L194 (55.2297, 3.4089) -> (57.745, 3.5199)
  line L195 (57.745, 3.5199) -> (59.0397, 3.5199)
  spline S147 degree 2 poles (59.0397, 3.5199) (60.4083, 3.5199) (60.4083, 5.4434) knots 0 0 0 1 1 1
  spline S148 degree 2 poles (60.4083, 5.4434) (60.4083, 9.7712) (57.856, 12.9524) knots 0 0 0 1 1 1
  spline S149 degree 2 poles (57.856, 12.9524) (57.0792, 11.6947) (57.0792, 11.1399) knots 0 0 0 1 1 1
  line L196 (57.0792, 11.1399) -> (57.856, 9.9562)
  line L197 (57.856, 9.9562) -> (57.856, 9.7343)
  line L198 (57.856, 9.7343) -> (57.745, 9.7343)
  spline S150 degree 2 poles (57.745, 9.7343) (53.935, 11.3988) (53.0843, 11.9907) knots 0 0 0 1 1 1
  line L199 (53.0843, 11.9907) -> (53.1582, 12.1016)
  line L200 (53.1582, 12.1016) -> (54.8228, 12.1016)
  spline S151 degree 2 poles (54.8228, 12.1016) (55.6736, 12.6935) (56.3764, 14.432) knots 0 0 0 1 1 1
  spline S152 degree 2 poles (56.3764, 14.432) (54.157, 16.2076) (48.8674, 18.242) knots 0 0 0 1 1 1
  spline S153 degree 2 poles (48.8674, 18.242) (48.1646, 18.8339) (43.5038, 19.9066) knots 0 0 0 1 1 1
  spline S154 degree 2 poles (43.5038, 19.9066) (41.1364, 20.8683) (38.991, 21.1643) knots 0 0 0 1 1 1
  line L201 (38.991, 21.1643) -> (38.732, 21.0903)
  line L202 (38.732, 21.0903) -> (32.2587, 21.8671)
  line L203 (32.2587, 21.8671) -> (31.9628, 21.7561)
  line L204 (31.9628, 21.7561) -> (31.6669, 21.8671)
  spline S155 degree 2 poles (31.6669, 21.8671) (27.7829, 21.4602) (25.8964, 20.6834) knots 0 0 0 1 1 1
  line L205 (25.8964, 20.6834) -> (19.4601, 19.0188)
  line L206 (19.4601, 19.0188) -> (19.4601, 19.2038)
  spline S156 degree 2 poles (19.4601, 19.2038) (27.7089, 22.4589) (29.8174, 22.4589) knots 0 0 0 1 1 1
  line L207 (29.8174, 22.4589) -> (31.297, 22.6439)
  line L208 (31.297, 22.6439) -> (31.7779, 22.5329)
  line L209 (31.7779, 22.5329) -> (33.3314, 22.5329)
  spline S157 degree 2 poles (33.3314, 22.5329) (43.1339, 22.5329) (51.1978, 19.3147) knots 0 0 0 1 1 1
  spline S158 degree 2 poles (51.1978, 19.3147) (52.1595, 19.3147) (57.1902, 17.0583) knots 0 0 0 1 1 1
  line L210 (57.1902, 17.0583) -> (57.2642, 16.9844)
  spline S159 degree 2 poles (57.2642, 16.9844) (57.3012, 16.7624) (57.856, 16.6884) knots 0 0 0 1 1 1
  line L211 (57.856, 16.6884) -> (57.856, 16.7624)
  line L212 (57.856, 16.7624) -> (58.4479, 17.8351)
  line L213 (58.4479, 17.8351) -> (57.2642, 19.0188)
  line L214 (57.2642, 19.0188) -> (57.2642, 19.1298)
  line L215 (57.2642, 19.1298) -> (57.3751, 19.1298)
  line L216 (57.3751, 19.1298) -> (61.666, 17.1693)
  line L217 (61.666, 17.1693) -> (61.666, 16.8734)
  line L218 (61.666, 16.8734) -> (60.7782, 17.0583)
  spline S160 degree 2 poles (60.7782, 17.0583) (60.0384, 17.0583) (59.4096, 15.5047) knots 0 0 0 1 1 1
  spline S161 degree 2 poles (59.4096, 15.5047) (62.3318, 13.2853) (63.1456, 11.2139) knots 0 0 0 1 1 1
  spline S162 degree 2 poles (63.1456, 11.2139) (65.1801, 8.6615) (65.1801, 4.0747) knots 0 0 0 1 1 1
  line L219 (65.1801, 4.0747) -> (65.1801, 3.7788)
  spline S163 degree 2 poles (65.1801, 3.7788) (65.1801, 2.8911) (64.5882, 1.2635) knots 0 0 0 1 1 1
  line L220 (64.5882, 1.2635) -> (63.4046, 1.4484)
  spline S164 degree 2 poles (63.4046, 1.4484) (62.0359, 1.2635) (62.0359, 0.3757) knots 0 0 0 1 1 1
  line L221 (62.0359, 0.3757) -> (62.0359, 0.0798)
  spline S165 degree 2 poles (62.0359, 0.0798) (62.0359, -0.882) (63.5155, -0.9929) knots 0 0 0 1 1 1
  spline S166 degree 2 poles (63.5155, -0.9929) (66.7707, -0.9929) (70.3587, 0.9676) knots 0 0 0 1 1 1
  spline S167 degree 2 poles (70.3587, 0.9676) (71.5424, 1.7444) (72.3932, 2.6321) knots 0 0 0 1 1 1
  line L222 (72.3932, 2.6321) -> (72.5042, 2.6321)
  line L223 (72.5042, 2.6321) -> (72.5042, 2.1143)
  spline S168 degree 2 poles (72.5042, 2.1143) (72.5042, 0.5237) (65.2911, -2.4725) knots 0 0 0 1 1 1
  line L224 (65.2911, -2.4725) -> (62.6647, -3.1384)
  spline S169 degree 2 poles (62.6647, -3.1384) (62.6647, -3.5453) (67.9174, -4.3221) knots 0 0 0 1 1 1
  line L225 (67.9174, -4.3221) -> (67.9174, -4.507)
  line L226 (67.9174, -4.507) -> (63.4046, -4.0261)
  line L227 (63.4046, -4.0261) -> (62.1469, -4.0261)
  spline S170 degree 2 poles (62.1469, -4.0261) (60.7413, -4.2851) (58.3369, -5.2098) knots 0 0 0 1 1 1
  line L228 (58.3369, -5.2098) -> (57.0792, -5.3948)
  line L229 (57.0792, -5.3948) -> (56.3024, -5.3948)
  spline S171 degree 2 poles (56.3024, -5.3948) (53.7501, -5.3948) (51.4197, -3.8412) knots 0 0 0 1 1 1
  line L230 (51.4197, -3.8412) -> (51.0128, -3.8412)
  line L231 (51.0128, -3.8412) -> (50.6429, -4.2111)
  line L232 (50.6429, -4.2111) -> (50.6429, -4.618)
  line L233 (50.6429, -4.618) -> (51.0128, -4.9879)
  line L234 (51.0128, -4.9879) -> (51.4197, -4.9879)
  line L235 (51.4197, -4.9879) -> (52.0115, -4.507)
  spline S172 degree 2 poles (52.0115, -4.507) (54.7118, -7.5032) (58.3369, -8.428) knots 0 0 0 1 1 1
  line L236 (58.3369, -8.428) -> (60.1864, -8.7239)
  line L237 (60.1864, -8.7239) -> (60.5933, -8.6129)
  line L238 (60.5933, -8.6129) -> (60.7043, -8.7239)
  line L239 (60.7043, -8.7239) -> (60.7043, -8.7979)
  spline S173 degree 2 poles (60.7043, -8.7979) (60.2604, -9.3897) (59.5206, -9.3897) knots 0 0 0 1 1 1
  line L240 (47.5357, -12.6819) -> (45.4643, -12.6819)
  spline S174 degree 2 poles (45.4643, -12.6819) (34.1452, -12.6819) (25.4525, -8.206) knots 0 0 0 1 1 1
  line L241 (25.4525, -8.206) -> (23.9729, -8.0951)
  spline S175 degree 2 poles (23.9729, -8.0951) (22.7522, -8.0951) (19.608, -8.6869) knots 0 0 0 1 1 1
  spline S176 degree 2 poles (19.608, -8.6869) (22.2344, -5.9496) (24.7497, -2.7315) knots 0 0 0 1 1 1
  line L242 (24.7497, -2.7315) -> (24.7497, -3.9891)
  spline S177 degree 2 poles (24.7497, -3.9891) (24.7497, -6.2455) (28.5967, -6.8374) knots 0 0 0 1 1 1
  spline S178 degree 2 poles (28.5967, -6.8374) (35.181, -5.0619) (35.4029, -4.692) knots 0 0 0 1 1 1
  spline S179 degree 2 poles (35.4029, -4.692) (36.6976, -4.1741) (36.6976, -3.3973) knots 0 0 0 1 1 1
  spline S180 degree 2 poles (36.6976, -3.3973) (36.6976, -2.4725) (35.5139, -2.1396) knots 0 0 0 1 1 1
  line L243 (35.5139, -2.1396) -> (32.1847, -3.3973)
  spline S181 degree 2 poles (32.1847, -3.3973) (29.1885, -2.5465) (25.1566, 0.1168) knots 0 0 0 1 1 1
  spline S182 degree 2 poles (25.1566, 0.1168) (21.5315, 2.928) (21.5315, 4.9995) knots 0 0 0 1 1 1
  line L244 (21.5315, 4.9995) -> (20.9767, 6.738)
  spline S183 degree 2 poles (20.9767, 6.738) (20.9767, 12.2866) (35.033, 18.8339) knots 0 0 0 1 1 1
  line L245 (35.033, 18.8339) -> (35.144, 18.8339)
  line L246 (35.144, 18.8339) -> (29.7434, 15.2458)
  line L247 (29.7434, 15.2458) -> (29.7434, 15.1348)
  line L248 (29.7434, 15.1348) -> (30.1503, 15.2458)
  spline S184 degree 2 poles (30.1503, 15.2458) (32.4067, 15.2458) (35.5139, 12.6195) knots 0 0 0 1 1 1
  spline S185 degree 2 poles (35.5139, 12.6195) (37.1784, 14.2471) (37.1784, 14.7649) knots 0 0 0 1 1 1
  line L249 (37.1784, 14.7649) -> (35.5879, 16.6884)
  line L250 (35.5879, 16.6884) -> (35.5879, 16.7994)
  line L251 (35.5879, 16.7994) -> (41.5063, 12.2496)
  line L252 (41.5063, 12.2496) -> (41.4323, 12.2496)
  spline S186 degree 2 poles (41.4323, 12.2496) (40.7665, 12.6565) (40.2486, 12.6565) knots 0 0 0 1 1 1
  line L253 (40.2486, 12.6565) -> (39.3609, 12.6565)
  line L254 (39.3609, 12.6565) -> (37.7333, 10.696)
  line L255 (37.7333, 10.696) -> (37.7333, 10.622)
  spline S187 degree 2 poles (37.7333, 10.622) (41.2474, 5.4434) (42.2461, 2.928) knots 0 0 0 1 1 1
  spline S188 degree 2 poles (42.2461, 2.928) (39.6568, 6.3681) (36.8455, 9.7343) knots 0 0 0 1 1 1
  spline S189 degree 2 poles (36.8455, 9.7343) (34.5891, 7.1079) (34.5891, 6.2942) knots 0 0 0 1 1 1
  line L256 (34.5891, 6.2942) -> (36.0317, 3.8528)
  line L257 (36.0317, 3.8528) -> (35.9578, 3.8528)
  line L258 (35.9578, 3.8528) -> (28.7816, 9.4753)
  line L259 (28.7816, 9.4753) -> (28.8556, 9.4753)
  line L260 (28.8556, 9.4753) -> (31.408, 8.4026)
  line L261 (31.408, 8.4026) -> (31.5189, 8.4026)
  spline S190 degree 2 poles (31.5189, 8.4026) (32.2217, 8.4026) (34.5151, 11.4358) knots 0 0 0 1 1 1
  spline S191 degree 2 poles (34.5151, 11.4358) (32.7766, 12.5085) (32.1108, 12.5085) knots 0 0 0 1 1 1
  line L262 (32.1108, 12.5085) -> (31.8888, 12.5085)
  spline S192 degree 2 poles (31.8888, 12.5085) (28.3747, 12.5085) (24.2688, 6.3681) knots 0 0 0 1 1 1
  line L263 (24.2688, 6.3681) -> (24.2688, 6.2572)
  spline S193 degree 2 poles (24.2688, 6.2572) (26.3033, 3.7048) (28.4857, 2.6321) knots 0 0 0 1 1 1
  spline S194 degree 2 poles (28.4857, 2.6321) (30.8161, 1.2635) (34.7371, 0.1908) knots 0 0 0 1 1 1
  spline S195 degree 2 poles (34.7371, 0.1908) (37.1414, -0.9559) (38.0662, -0.9559) knots 0 0 0 1 1 1
  line L264 (38.0662, -0.9559) -> (39.028, -0.9559)
  spline S196 degree 2 poles (39.028, -0.9559) (40.5815, -0.9559) (43.2079, 0.4127) knots 0 0 0 1 1 1
  spline S197 degree 2 poles (43.2079, 0.4127) (40.5076, -2.1026) (40.5076, -2.3246) knots 0 0 0 1 1 1
  line L265 (40.5076, -2.3246) -> (40.5076, -2.4355)
  line L266 (40.5076, -2.4355) -> (40.5815, -2.4355)
  spline S198 degree 2 poles (40.5815, -2.4355) (42.4311, -1.8437) (46.0561, 1.0785) knots 0 0 0 1 1 1
  spline S199 degree 2 poles (46.0561, 1.0785) (47.2398, 1.4854) (49.9771, 4.1117) knots 0 0 0 1 1 1
  spline S200 degree 2 poles (49.9771, 4.1117) (50.7169, 5.3324) (51.5307, 6.1462) knots 0 0 0 1 1 1
  line L267 (51.5307, 6.1462) -> (54.6379, 11.7317)
  spline S201 degree 2 poles (54.6379, 11.7317) (54.6379, 12.2126) (56.0065, 13.7662) knots 0 0 0 1 1 1
  line L268 (56.0065, 13.7662) -> (56.1175, 13.7662)
  line L269 (56.1175, 13.7662) -> (56.1175, 13.6922)
  spline S202 degree 2 poles (56.1175, 13.6922) (52.2705, 4.7036) (50.458, 3.4459) knots 0 0 0 1 1 1
  spline S203 degree 2 poles (50.458, 3.4459) (44.3546, -2.3986) (41.3953, -3.8042) knots 0 0 0 1 1 1
  spline S204 degree 2 poles (41.3953, -3.8042) (37.8443, -5.9496) (32.1108, -8.391) knots 0 0 0 1 1 1
  line L270 (32.1108, -8.391) -> (31.297, -8.5759)
  spline S205 degree 2 poles (31.297, -8.5759) (31.371, -8.7979) (34.5151, -9.6487) knots 0 0 0 1 1 1
  spline S206 degree 2 poles (34.5151, -9.6487) (38.4361, -11.4242) (42.764, -11.4242) knots 0 0 0 1 1 1
  spline S207 degree 2 poles (42.764, -11.4242) (43.0969, -11.6831) (45.5752, -11.9051) knots 0 0 0 1 1 1
  line L271 (45.5752, -11.9051) -> (47.1288, -11.9051)
  spline S208 degree 2 poles (47.1288, -11.9051) (50.8279, -11.4242) (52.7883, -10.4624) knots 0 0 0 1 1 1
  spline S209 degree 2 poles (52.7883, -10.4624) (55.2297, -9.8706) (57.4861, -8.9828) knots 0 0 0 1 1 1
  line L272 (57.4861, -8.9828) -> (58.6698, -8.6869)
  line L273 (58.6698, -8.6869) -> (58.7808, -8.7979)
  line L274 (58.7808, -8.7979) -> (58.7808, -8.8719)
  spline S210 degree 2 poles (58.7808, -8.8719) (50.7539, -12.6079) (48.3125, -12.6079) knots 0 0 0 1 1 1
  line L275 (48.3125, -12.6079) -> (47.5357, -12.6819)
  point P0 (162.56, 10.16)
  point P1 (151.5154, -15.0492)
  constraints: 1 other